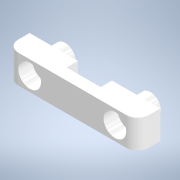
# Autodesk Inventor part: ZTopCable
Saved by Autodesk Inventor 2020 (Build 240168000, 168)
## iProperties
Created: 2022-05-19
Part Number: ZTopCable
Material: Tworzywo sztuczne ABS
Document SubType Name: Modeling
Designer: mikoma
Density: 1.06 g/cm^3
Appearance: Gładki — biały
Mass: 2.95498 g
Surface Area: 23.6375 cm^2
Volume: 2.78772 cm^3
Author: mikoma
Autodesk Inventor part; units mm, degrees
ref_plane "YZ Plane" through (0, 0, 0) normal (1, 0, 0) x (0, 1, 0)
ref_plane "XZ Plane" through (0, 0, 0) normal (0, 1, 0) x (-1, 0, 0)
ref_plane "XY Plane" through (0, 0, 0) normal (0, 0, 1) x (1, 0, 0)
sketch "Szkic1" plane through (0, 0, 0) normal (0, 0, 1) x (1, 0, 0)
  line L0 (-23, -5) -> (23, -5)
  line L1 (23, -5) -> (23, 5)
  line L2 (23, 5) -> (-23, 5)
  line L3 (-23, 5) -> (-23, -5)
  line L4 (-23, -5) -> (23, 5) construction
  line L5 (23, -5) -> (-23, 5) construction
  circle A0 centre (-15, 0) radius 3.75
  circle A1 centre (-15, 0) radius 2.25
  circle A2 centre (15, 0) radius 3.75
  circle A3 centre (15, 0) radius 2.25
  line L6 (-6, -5) -> (6, -5)
  line L7 (6, -5) -> (6, 5)
  line L8 (6, 5) -> (-6, 5)
  line L9 (-6, 5) -> (-6, -5)
  line L10 (-6, -5) -> (6, 5) construction
  line L11 (6, -5) -> (-6, 5) construction
  circle A4 centre (-15, 0) radius 4
  circle A5 centre (15, 0) radius 4
  point P0 (0, 0)
  point P1 (0, 0)
  dimension "d1" = 10
  dimension "d3" = 7.5
  dimension "d4" = 4.5
  dimension "d6" = 15
  dimension "d7" = 15
  dimension "d8" = 8
  dimension "d9" = 6
  dimension "d18" = 8
  dimension "d19" = 8
  constraints: 24 end point, 6 centre point, 5 midpoint, 4 coincident, 4 parallel, 2 equal radius, 2 horizontal, 2 horizontal alignment, 2 perpendicular, 1 point on line
  measures "d1" distance of L0.end L1.end
  measures "d3" diameter of A0
  measures "d4" diameter of A1
  measures "d6" distance of point (0, 0) A1.centre
  measures "d7" distance of A2.centre point (0, 0)
  measures "d8" distance from line of L3 A0.centre
  measures "d9" distance from line of L9 point (0, 0)
  measures "d18" diameter of A5
  measures "d19" diameter of A4
extrude "Wyciągnięcie proste1" add sketch "Szkic1" along normal blind 8 contours L3 L2 L9 L0 | L9 L2 L7 L0 | L7 L2 L1 L0 | A0 | A1 | A2 | A3 | A4 | A5
extrude "Wyciągnięcie proste2" cut sketch "Szkic1" along normal blind 4 contours L9 L2 L7 L0
extrude "Wyciągnięcie proste3" cut sketch "Szkic1" along normal through all contours A1 | A3
extrude "Wyciągnięcie proste4" add sketch "Szkic1" against normal blind 4.5 contours A0 | A2
extrude "Wyciągnięcie proste5" cut sketch "Szkic1" against normal blind 5 from surface at 8 contours A0 | A1 | A2 | A3 | A4 | A5
fillet "Zaokrąglenie1" radius 4 2 edges at (23, 0, 8) (-23, 0, 8)
